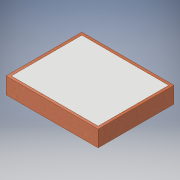
# Autodesk Inventor part: OpticalDeviceLookThroughPart
Saved by Autodesk Inventor 2017 (Build 210142000, 142)
## iProperties
Created: 2019-04-03
Part Number: OpticalDeviceLookThroughPart
Material: Glass
Document SubType Name: Modeling
Designer: Sharat
Density: 2.18 g/cm^3
Appearance: Walnut - Natural Polished
Author: Sharat
Autodesk Inventor part; units mm, degrees
ref_plane "YZ Plane" through (0, 0, 0) normal (1, 0, 0) x (0, 1, 0)
ref_plane "XZ Plane" through (0, 0, 0) normal (0, 1, 0) x (-1, 0, 0)
ref_plane "XY Plane" through (0, 0, 0) normal (0, 0, 1) x (1, 0, 0)
sketch "Sketch1" plane through (0, 0, 0) normal (0, 1, 0) x (-1, 0, 0)
  line L0 (0, 0) -> (170, 0)
  line L1 (170, 0) -> (170, -140)
  line L2 (170, -140) -> (0, -140)
  line L3 (0, -140) -> (0, 0)
  line L4 (165.2375, -4.7625) -> (4.7625, -4.7625)
  line L5 (4.7625, -4.7625) -> (4.7625, -135.2375)
  line L6 (4.7625, -135.2375) -> (165.2375, -135.2375)
  line L7 (165.2375, -135.2375) -> (165.2375, -4.7625)
  dimension "d0" = 170
  dimension "d1" = 140
  dimension "d2" = 4.7625
  dimension "d3" = 4.7625
  dimension "d4" = 4.7625
  dimension "d5" = 4.7625
  dimension "d6" = 4.7625
  constraints: 16 end point, 4 parallel, 2 horizontal, 1 perpendicular, 1 vertical
  measures "d0" distance of L1.end L2.end
  measures "d1" distance of L0.end L1.end
  measures "d2" distance between parallel lines of L0 L4
  measures "d3" distance from line of L1 L4.start
  measures "d4" distance from line of L3 L4.end
  measures "d5" distance between parallel lines of L2 L6
  measures "d6" distance between parallel lines of L3 L5
extrude "Extrusion1" add sketch "Sketch1" along normal blind 30
sketch "Sketch2" plane through (0, 30, 0) normal (0, 1, 0) x (1, 0, 0)
  line L0 (-4.7625, 4.7625) -> (-165.2375, 4.7625) projected
  line L1 (-165.2375, 4.7625) -> (-4.7625, 4.7625)
  line L2 (-4.7625, 4.7625) -> (-4.7625, 135.2375)
  line L3 (-4.7625, 135.2375) -> (-165.2375, 135.2375)
  line L4 (-165.2375, 135.2375) -> (-165.2375, 4.7625)
  point P0 (0, 0)
  constraints: 8 end point, 2 parallel, 1 horizontal, 1 perpendicular
extrude "Extrusion2" add sketch "Sketch2" against normal blind 12.7
sketch "Sketch3" plane through (0, 30, 0) normal (0, 1, 0) x (1, 0, 0)
  line L0 (-165.2375, 135.2375) -> (-165.2375, 4.7625) projected
  line L1 (-4.7625, 4.7625) -> (-4.7625, 135.2375) projected
  line L2 (-165.2375, 4.7625) -> (-4.7625, 4.7625)
  line L3 (-4.7625, 4.7625) -> (-4.7625, 135.2375)
  line L4 (-4.7625, 135.2375) -> (-165.2375, 135.2375)
  line L5 (-165.2375, 135.2375) -> (-165.2375, 4.7625)
  point P0 (0, 0)
  constraints: 8 end point, 2 parallel, 1 horizontal, 1 perpendicular
extrude "Extrusion3" add sketch "Sketch3" along normal blind 0.0254
body "Solid1"
